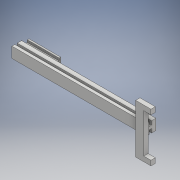
# Autodesk Inventor part: trilho sem cremalheira
Saved by Autodesk Inventor 2018 (Build 220112000, 112)
## iProperties
Created: 2018-06-04
Part Number: trilho sem cremalheira
Material: Genérico
Document SubType Name: Modeling
Designer: Ernandes
Density: 1 g/cm^3
Appearance: Padrão
Author: Ernandes
Autodesk Inventor part; units mm, degrees
ref_plane "YZ Plane" through (0, 0, 0) normal (1, 0, 0) x (0, 1, 0)
ref_plane "XZ Plane" through (0, 0, 0) normal (0, 1, 0) x (-1, 0, 0)
ref_plane "XY Plane" through (0, 0, 0) normal (0, 0, 1) x (1, 0, 0)
sketch "Esboço1" plane through (0, 0, 0) normal (0, 1, 0) x (-1, 0, 0)
  line L0 (0, 0) -> (0, -18.5)
  line L1 (0, 0) -> (232.5, 0)
  line L2 (232.5, 0) -> (232.5, -18.5)
  line L3 (232.5, -18.5) -> (0, -18.5)
  dimension "d0" = 18.5
  dimension "d1" = 232.5
  constraints: 8 end point, 2 perpendicular, 1 horizontal, 1 vertical
  measures "d0" distance of L0.start L0.end
  measures "d1" distance of L0.start L1.end
extrude "Extrusão1" add sketch "Esboço1" along normal blind 5
sketch "Esboço2" plane through (0, 5, 0) normal (0, 1, 0) x (1, 0, 0)
  line L0 (0, 0) -> (0, 9.25)
  line L1 (0, 0) -> (0, 18.5) projected
  line L2 (0, 9.25) -> (0, 11.75)
  line L3 (0, 11.75) -> (0, 6.75)
  line L4 (0, 6.75) -> (-232.5, 6.75)
  line L5 (-232.5, 18.5) -> (-232.5, 0) projected
  line L6 (-232.5, 6.75) -> (-232.5, 11.75)
  line L7 (-232.5, 11.75) -> (0, 11.75)
  dimension "d4" = 2.5
  dimension "d5" = 5
  constraints: 12 end point, 3 point on line, 2 perpendicular, 1 midpoint, 1 vertical
  measures "d4" distance of L0.end L2.end
  measures "d5" distance of L2.end L3.end
extrude "Extrusão2" add sketch "Esboço2" along normal blind 4
sketch "Esboço3" plane through (0, 9, 0) normal (0, 1, 0) x (1, 0, 0)
  line L0 (-232.5, 6.75) -> (0, 6.75) projected
  line L1 (0, 0) -> (0, 18.5) projected
  line L2 (0, 6.75) -> (0, 18.5)
  line L3 (0, 18.5) -> (0, 0)
  line L4 (0, 0) -> (-232.5, 0)
  line L5 (0, 18.5) -> (-232.5, 18.5) projected
  line L6 (-232.5, 18.5) -> (-232.5, 11.75) projected
  line L7 (-232.5, 0) -> (-232.5, 18.5)
  line L8 (-232.5, 18.5) -> (0, 18.5)
  constraints: 10 end point, 2 equal length, 2 perpendicular, 1 vertical
extrude "Extrusão3" add sketch "Esboço3" along normal blind 7.5
sketch "Esboço4" plane through (0, 0, 0) normal (0, -1, 0) x (1, 0, 0)
  line L0 (-232.5, 0) -> (0, 0) projected
  line L1 (-11, -9.25) -> (-11, -51.75)
  line L2 (-11, -51.75) -> (15.5, -51.75)
  line L3 (15.5, -51.75) -> (15.5, -43.25)
  line L4 (15.5, -43.25) -> (3, -43.25)
  line L5 (-11, -9.25) -> (-11, 33.25)
  line L6 (-11, 33.25) -> (15.5, 33.25)
  line L7 (15.5, 33.25) -> (15.5, 24.75)
  line L8 (15.5, 24.75) -> (3, 24.75)
  line L9 (3, 24.75) -> (3, -43.25)
  dimension "d12" = 42.5
  dimension "d14" = 26.5
  dimension "d15" = 8.5
  dimension "d17" = 42.5
  dimension "d18" = 8.5
  constraints: 18 end point, 3 perpendicular, 2 horizontal, 2 vertical, 1 parallel
  measures "d12" distance of L1.start L1.end
  measures "d14" distance of L1.end L2.end
  measures "d15" distance of L2.end L3.end
  measures "d17" distance of L1.start L5.end
  measures "d18" distance of L6.end L7.end
extrude "Extrusão4" add sketch "Esboço4" along normal blind 7.5
sketch "Esboço5" plane through (0, 16.5, 0) normal (0, 1, 0) x (1, 0, 0)
  line L0 (0, 18.5) -> (-232.5, 18.5) projected
  line L1 (-232.5, 18.5) -> (-232.5, 0) projected
  line L2 (-232.5, 9.25) -> (-232.5, 10.75)
  line L3 (-232.5, 10.75) -> (-232.5, 7.75)
  line L4 (-232.5, 7.75) -> (-177.5, 7.75)
  line L5 (-177.5, 7.75) -> (-177.5, 10.75)
  line L6 (0, 11.75) -> (-232.5, 11.75) projected
  line L7 (-177.5, 10.75) -> (-232.5, 10.75)
  point P0 (0, 0)
  dimension "d21" = 1.5
  dimension "d22" = 3
  dimension "d23" = 55
  dimension "d24" = 3
  constraints: 10 end point, 2 perpendicular, 2 point on line, 1 midpoint
  measures "d21" distance of L2.start L2.end
  measures "d22" distance of L2.end L3.end
  measures "d23" distance of L3.end L4.end
  measures "d24" distance of L4.end L5.end
extrude "Extrusão5" add sketch "Esboço5" along normal blind 10
sketch "Esboço6" plane through (0, 26.5, 0) normal (0, 1, 0) x (1, 0, 0)
  line L0 (-232.5, 10.75) -> (-232.5, 7.75) projected
  line L1 (-232.5, 9.25) -> (-232.5, 14.75)
  line L2 (-232.5, 14.75) -> (-232.5, 3.75)
  line L3 (-232.5, 6.75) -> (-232.5, 0) projected
  line L4 (-232.5, 3.75) -> (-177.5, 3.75)
  line L5 (-177.5, 3.75) -> (-177.5, 14.75)
  line L6 (-177.5, 14.75) -> (-232.5, 14.75)
  line L7 (0, 18.5) -> (-232.5, 18.5) projected
  point P0 (0, 0)
  dimension "d27" = 5.5
  dimension "d28" = 11
  dimension "d29" = 55
  constraints: 10 end point, 2 perpendicular, 1 collinear, 1 midpoint, 1 parallel, 1 point on line
  measures "d27" distance of L1.start L1.end
  measures "d28" distance of L1.end L2.end
  measures "d29" distance of L2.end L4.end
extrude "Extrusão6" add sketch "Esboço6" along normal blind 3
